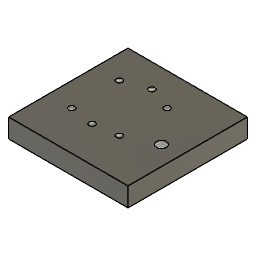
Y Axis End (Autodesk Fusion 360 design; units mm, degrees)
Autodesk Fusion 360 part; units mm, degrees
note: some values were not read from the file. Set by a fixed rule: which sketch regions a step uses; the direction of a hole.
sketch "Sketch1" plane through (0, 0, 0) normal (0, 0, 1) x (1, 0, 0)
  line L0 (20, -25) -> (-20, -25)
  line L1 (-20, -25) -> (-20, 25)
  line L2 (-20, 25) -> (20, 25)
  line L3 (20, 25) -> (20, -25)
  line L4 (20, -25) -> (-20, 25) construction
  line L5 (-20, -25) -> (20, 25) construction
  line L6 (20, -18.5) -> (20, 12.5)
  line L7 (20, 25) -> (30, 25)
  line L8 (30, 25) -> (30, -25)
  line L9 (30, -25) -> (20, -25)
  line L10 (20, -25) -> (20, 25)
  point P0 (-10, 11.4115)
  point P1 (10, 11.4115)
  point P2 (10, -8.5885)
  point P3 (-10, -8.5885)
  point P4 (0, 15)
  point P5 (0, -10)
  point P6 (22, -3)
  dimension "d19" = 40
  dimension "d20" = 50
  dimension "d22" = 20
  dimension "d23" = 20
  dimension "d25" = 25
  dimension "d34" = 31
  dimension "d41" = 22
  dimension "d42" = 10
  constraint horizontal L0
  constraint perpendicular L0 L1
  constraint parallel L0 L2
  constraint parallel L1 L3
  constraint coincident L4 origin
  constraint coincident L5 origin
  constraint vertical L6
  constraint coincident L3 L6.end
  constraint horizontal L7
  constraint vertical L8
  constraint horizontal L9
  constraint vertical L10
  measures "d19" distance of L1.end L2.end
  measures "d20" distance of L0.end L1.end
  measures "d22" distance of P0 P1
  measures "d23" distance of P0 P3
  measures "d25" distance of P4 P5
  measures "d34" distance of L6.end L6.start
  measures "d41" horizontal distance of origin P6
  measures "d42" distance of L2.end L7.end
extrude "Extrude2" add sketch "Sketch1" along normal blind 8
hole "Hole3" at (0, -10, 0) at (10, -8.5885, 0) at (10, 11.4115, 0) at (0, 15, 0) at (-10, 11.4115, 0) at (-10, -8.5885, 0) direction (0, 0, 1) diameter 2.529 depth 15 tip angle 118
thread "Thread3" "ISO Metric profile 3.0 M3x0.5 M3x0.5 6H" thread offset 0 thread depth 7.4
hole "Hole4" at (22, -3, 0) direction (0, 0, 1) diameter 4.234 depth 20 tip angle 118
thread "Thread4" "ISO Metric profile 5.0 M5x0.8 M5x0.8 6H" thread offset 0 thread depth 7.4
